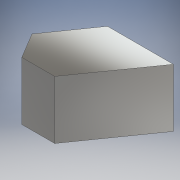
# Autodesk Inventor part: metal_shielding
Saved by Autodesk Inventor 2018 (Build 220112000, 112)
## iProperties
Created: 2019-03-10
Part Number: metal_shielding
Material: Generic
Document SubType Name: Modeling
Designer: ZEUSLAP
Density: 1 g/cm^3
Appearance: Default
Author: ZEUSLAP
Autodesk Inventor part; units mm, degrees
ref_plane "YZ Plane" through (0, 0, 0) normal (1, 0, 0) x (0, 1, 0)
ref_plane "XZ Plane" through (0, 0, 0) normal (0, 1, 0) x (-1, 0, 0)
ref_plane "XY Plane" through (0, 0, 0) normal (0, 0, 1) x (1, 0, 0)
sketch "Sketch1" plane through (0, 0, 0) normal (0, 0, 1) x (1, 0, 0)
  line L0 (0, 0) -> (-17, 0)
  line L1 (-17, 0) -> (-25.0301, -11.4681)
  line L2 (0, 0) -> (-12.6187, -18.0213)
  line L3 (0, 0) -> (22, 0) construction
  line L4 (-12.6187, -18.0213) -> (-21.1187, -18.0213)
  line L5 (-21.1187, -18.0213) -> (-25.0301, -11.4681)
  dimension "d40" = 17
  dimension "d41" = 14
  dimension "d42" = 125
  dimension "d43" = 22
  dimension "d44" = 125
  dimension "d45" = 8.5
  constraints: 12 end point, 3 horizontal, 1 equal length
  measures "d40" distance of L0.start L0.end
  measures "d41" distance of L0.end L1.end
  measures "d42" angle of L1 L0
  measures "d43" distance of L0.start L2.end
  measures "d44" angle of L2 L3
  measures "d45" distance of L2.end L4.end
extrude "Extrusion1" add sketch "Sketch1" along normal blind 15
shell "Shell1" thickness 0.5 removed faces 2 at (-5.6667, 0, 5) at (-9.8729, -6.0071, 0)
body "Solid1"
